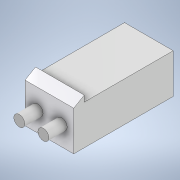
# Autodesk Inventor part: conector_4pines
Saved by Autodesk Inventor 2020 (Build 240168000, 168)
## iProperties
Created: 2021-10-19
Part Number: conector_4pines
Material: Genérico
Document SubType Name: Modeling
Designer: DANIEL
Density: 1 g/cm^3
Appearance: Valor por defecto
Author: DANIEL
Autodesk Inventor part; units mm, degrees
ref_plane "YZ Plane" through (0, 0, 0) normal (1, 0, 0) x (0, 1, 0)
ref_plane "XZ Plane" through (0, 0, 0) normal (0, 1, 0) x (-1, 0, 0)
ref_plane "XY Plane" through (0, 0, 0) normal (0, 0, 1) x (1, 0, 0)
sketch "Boceto1" plane through (0, 0, 0) normal (0, 1, 0) x (-1, 0, 0)
  line L0 (8, 8.175) -> (-8, 8.175)
  line L1 (-8, 8.175) -> (-8, -8.175)
  line L2 (-8, -8.175) -> (8, -8.175)
  line L3 (8, -8.175) -> (8, 8.175)
  point P0 (0, 0)
  dimension "d0" = 16.35
  dimension "d1" = 16
  dimension "d2" = 8
  dimension "d3" = 8.175
  constraints: 8 end point, 2 parallel, 1 horizontal, 1 perpendicular
  measures "d0" distance between parallel lines of L2 L0
  measures "d1" distance between parallel lines of L1 L3
  measures "d2" distance from line of L3 point (0, 0)
  measures "d3" distance from line of L0 point (0, 0)
extrude "Extrusión1" add sketch "Boceto1" along normal mid plane 6.5
sketch "Boceto2" plane through (8, -3.25, -8.175) normal (1, 0, 0) x (0, 0, -1)
  line L0 (0, 0) -> (0, 6.5) projected
  line L1 (-16.35, 6.5) -> (0, 6.5) projected
  line L2 (-16.35, 0) -> (-16.35, 6.5) projected
  line L3 (0, 0) -> (-16.35, 0) projected
  line L4 (0, 6.5) -> (-16.35, 6.5) projected
  line L5 (-16.35, 6.5) -> (-14.6179, 7.5)
  line L6 (-14.6179, 7.5) -> (-14.6179, 6.5)
  line L7 (-16.35, 6.5) -> (-14.6179, 6.5)
  point P0 (-8.175, 3.25)
  dimension "d6" = 7.5
  dimension "d7" = 60
  constraints: 6 end point, 1 collinear, 1 perpendicular, 1 point on line
  measures "d6" distance from line of L5.end L3
  measures "d7" angle of L5 L6
extrude "Extrusión2" add sketch "Boceto2" against normal blind 16 contours L1 L5 L6
sketch "Boceto3" plane through (-8, -3.25, 8.175) normal (0, 0, 1) x (1, 0, 0)
  line L0 (16, 0) -> (16, 6.5) projected
  line L1 (0, 6.5) -> (16, 6.5) projected
  line L2 (0, 0) -> (0, 6.5) projected
  line L3 (16, 0) -> (0, 0) projected
  circle A0 centre (13.94, 3.25) radius 0.9
  circle A1 centre (9.98, 3.25) radius 0.9
  circle A2 centre (6.02, 3.25) radius 0.9
  circle A3 centre (2.06, 3.25) radius 0.9
  point P0 (8, 3.25)
  dimension "d10" = 3.25
  dimension "P" = 3.96
  dimension "d12" = 3.96
  dimension "d13" = 3.96
  dimension "d14" = 2.06
  dimension "d15" = 1.8
  dimension "d16" = 1.8
  dimension "d17" = 1.8
  dimension "d18" = 1.8
  constraints: 4 centre point, 4 coincident, 3 horizontal alignment
  measures "d10" distance from line of L1 point (13.94, 3.25)
  measures "P" distance of point (9.98, 3.25) point (13.94, 3.25)
  measures "d12" distance of point (9.98, 3.25) point (6.02, 3.25)
  measures "d13" distance of point (6.02, 3.25) point (2.06, 3.25)
  measures "d14" distance from line of L2 point (2.06, 3.25)
  measures "d15" diameter of A0
  measures "d16" diameter of A1
  measures "d17" diameter of A2
  measures "d18" diameter of A3
extrude "Extrusión3" add sketch "Boceto3" along normal blind 3 contours A0 | A1 | A2 | A3
sketch "Boceto4" plane through (-8, -3.25, 8.175) normal (0, 0, 1) x (1, 0, 0)
  circle A0 centre (6.02, 3.25) radius 0.9 projected
  circle A1 centre (9.98, 3.25) radius 0.9 projected
  circle A2 centre (2.06, 3.25) radius 0.9 projected
  circle A3 centre (13.94, 3.25) radius 0.9 projected
  line L0 (16, 0) -> (16, 6.5) projected
  line L1 (0, 6.5) -> (16, 6.5) projected
  line L2 (0, 0) -> (0, 6.5) projected
  line L3 (16, 0) -> (0, 0) projected
  line L4 (8, 0) -> (16.3652, 0)
  line L5 (16.3652, 0) -> (16.3652, 8.0001)
  line L6 (16.3652, 8.0001) -> (8, 8.0001)
  line L7 (8, 8.0001) -> (8, 0)
  point P0 (8, 3.25)
  constraints: 8 end point, 2 parallel, 1 horizontal, 1 midpoint, 1 perpendicular
extrude "Extrusión4" cut sketch "Boceto4" against normal mid plane 40 contours A1 | A3 | L3 L7 L1 L0 | L0 L1 L7 L6 L5 L4
equation "\"d12\" = P"
equation "\"d13\" = P"
